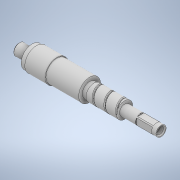
# Autodesk Inventor part: 75. Шестерня спидометра ведомая
Saved by Autodesk Inventor 2021 (Build 250183000, 183)
## iProperties
Created: 2021-03-27
Part Number: 75. Шестерня спидометра ведомая
Material: Типовые
Document SubType Name: Modeling
Designer: Данил
Density: 1 g/cm^3
Appearance: По умолчанию
Author: Данил
Autodesk Inventor part; units mm, degrees
ref_plane "YZ Plane" through (0, 0, 0) normal (1, 0, 0) x (0, 1, 0)
ref_plane "XZ Plane" through (0, 0, 0) normal (0, 1, 0) x (-1, 0, 0)
ref_plane "XY Plane" through (0, 0, 0) normal (0, 0, 1) x (1, 0, 0)
sketch "Эскиз1" plane through (0, 0, 0) normal (0, 0, 1) x (1, 0, 0)
  line L0 (-48.75, 0) -> (48.75, 0)
  line L1 (48.75, 0) -> (48.75, -3.5)
  line L2 (48.75, -3.5) -> (23.75, -3.5)
  line L3 (23.75, -3.5) -> (23.75, -5.5)
  line L4 (23.75, -5.5) -> (2.75, -5.5)
  line L5 (2.75, -5.5) -> (2.75, -5)
  line L6 (2.75, -5) -> (-0.25, -5)
  line L7 (-0.25, -5) -> (-0.25, -7.5)
  line L8 (-0.25, -7.5) -> (-22.75, -7.5)
  line L9 (-22.75, -7.5) -> (-22.75, -10.55)
  line L10 (-22.75, -10.55) -> (-36.75, -10.55)
  line L11 (-36.75, -10.55) -> (-36.75, -7.5)
  line L12 (-36.75, -7.5) -> (-39.75, -7.5)
  line L13 (-39.75, -7.5) -> (-39.75, -3.5)
  line L14 (-39.75, -3.5) -> (-41.25, -3.5)
  line L15 (-41.25, -3.5) -> (-41.25, -4)
  line L16 (-41.25, -4) -> (-48.25, -4)
  line L17 (-48.75, -3.5) -> (-48.75, 0)
  line L18 (-48.25, -4) -> (-48.75, -3.5)
  point P0 (0, 0)
  point P1 (0, 0)
  point P2 (-48.75, -4)
  dimension "d0" = 97.5
  dimension "d1" = 7
  dimension "d2" = 25
  dimension "d3" = 11
  dimension "d4" = 10
  dimension "d5" = 3
  dimension "d6" = 15
  dimension "d7" = 24
  dimension "d8" = 14
  dimension "d9" = 15
  dimension "d10" = 0.5
  dimension "d11" = 45
  dimension "d12" = 8
  dimension "d13" = 7
  dimension "d14" = 1.5
  dimension "d15" = 9
  dimension "d16" = 3
  dimension "d17" = 21.1
  constraints: 38 end point, 10 perpendicular, 6 vertical, 3 point on line, 2 coincident, 1 horizontal, 1 midpoint, 1 parallel
  measures "d0" distance of L0.start L0.end
  measures "d1" diameter of L2 L0
  measures "d2" horizontal distance of L0.end L2.end
  measures "d3" diameter of L4 L0
  measures "d4" diameter of L6 L0
  measures "d5" distance of L5.end L6.end
  measures "d6" diameter of L8 L0
  measures "d7" distance between parallel lines of L7 L3
  measures "d8" distance of L9.end L10.end
  measures "d9" diameter of L12 L0
  measures "d10" distance of L16.end point (-48.75, -4)
  measures "d11" angle of L16 L18
  measures "d12" diameter of L16 L0
  measures "d13" diameter of L14 L0
  measures "d14" distance of L13.end L14.end
  measures "d15" distance from line of L0.start L13
  measures "d16" distance of L11.end L12.end
  measures "d17" diameter of L10 L0
revolve "Вращение1" add sketch "Эскиз1" angle 360 about axis through (-48.75, 0, 0) along (1, 0, 0)
sketch "Эскиз2" plane through (0, 0, 0) normal (0, 0, 1) x (1, 0, 0)
  line L0 (48.75, 3.5) -> (23.75, 3.5) projected
  line L1 (48.75, 3.5) -> (48.75, -3.5) projected
  line L2 (48.75, 3.5) -> (45.85, 3.5)
  line L3 (45.65, 2.75) -> (34.85, 2.75)
  line L4 (34.75, 2.85) -> (34.75, 3.4)
  line L5 (45.75, 2.85) -> (45.75, 3.4)
  line L6 (34.65, 3.5) -> (23.75, 3.5)
  line L7 (23.75, 5.5) -> (23.75, -5.5) projected
  arc A0 (34.75, 3.4) -> (34.65, 3.5) centre (34.65, 3.4) ccw
  arc A1 (34.75, 2.85) -> (34.85, 2.75) centre (34.85, 2.85) ccw
  arc A2 (45.65, 2.75) -> (45.75, 2.85) centre (45.65, 2.85) ccw
  arc A3 (45.85, 3.5) -> (45.75, 3.4) centre (45.85, 3.4) ccw
  line L8 (23.75, 3.5) -> (48.75, 3.5)
  point P0 (0, 0)
  point P1 (45.75, 3.5)
  point P2 (45.75, 2.75)
  point P3 (34.75, 2.75)
  point P4 (34.75, 3.5)
  dimension "d19" = 3
  dimension "d20" = 14
  dimension "d21" = 0.75
  dimension "d22" = 0.1
  dimension "d23" = 0.1
  constraints: 12 end point, 10 point on line, 8 point on circle, 8 tangent, 4 centre point, 2 equal radius, 2 perpendicular, 1 collinear, 1 horizontal, 1 vertical
  measures "d19" distance of L0.start point (45.75, 3.5)
  measures "d20" distance from line of point (34.75, 2.75) L1
  measures "d21" distance of point (45.75, 2.75) point (45.75, 3.5)
  measures "d22" radius of A0
  measures "d23" radius of A2
extrude "Выдавливание1" cut sketch "Эскиз2" against normal through all both and the other way through all
mirror "Зеркальное отражение1" about plane through (0, 0, 0) normal (0, 1, 0) of "Выдавливание1"
pattern_circular "Круговой массив1" count 2 over 90 about axis through (36.25, 0, 0) along (-1, 0, 0) of "Выдавливание1"
mirror "Зеркальное отражение2" about plane through (0, 0, 0) normal (0, 0, 1) of "Круговой массив1"
ref_plane "РабПлоскость1" through (23.75, 0, 5.5) normal (0.2255336, -0.9742354, 0) x (0.9742354, 0.2255336, 0)
sketch "Эскиз3" plane through (23.75, 0, 5.5) normal (0.2255336, -0.9742354, 0) x (0.9742354, 0.2255336, 0)
  line L0 (-0.6243, 0) -> (-0.2121, -0.4121)
  line L1 (0.6243, 0) -> (0.2121, -0.4121)
  arc A0 (-0.2121, -0.4121) -> (0.2121, -0.4121) centre (0, -0.2) ccw
  line L2 (-0.6243, 0) -> (0.6243, 0)
  point P0 (-23.1381, -5.5)
  point P1 (0, 0)
  point P2 (0, -0.5)
  dimension "d37" = 90
  dimension "d38" = 0.5
  dimension "d39" = 0.5
  dimension "d40" = 0.3
  constraints: 6 end point, 3 point on circle, 2 tangent, 2 vertical alignment, 1 centre point, 1 horizontal alignment
  measures "d37" angle of L0 L1
  measures "d38" vertical distance of point (0, -0.5) L1.start
  measures "d39" vertical distance of point (0, -0.5) L0.start
  measures "d40" radius of A0
sketch3d "3D эскиз1"
  helix H0 starts at (3.75, 0, -5.5) axis through (3.75, 0, 0) along (1, 0, 0) pitch 8 turns 2.5 hand right
sweep "Сдвиг1" cut profiles "Эскиз3" path "3D эскиз1"
sketch "Эскиз4" plane through (48.75, 0, 0) normal (1, 0, 0) x (0, 0, -1)
  circle A0 centre (0, 0) radius 3.5 projected
  point P0 (0, 0)
hole "Отверстие1" at (48.75, 0, 0) direction (-1, 0, 0) diameter 4 depth 27 tip angle 120 counterbore diameter 5 counterbore depth 3
chamfer "Фаска1" distance 0.5 angle 60 1 edges at (48.75, 0, 2.5) measured on face at (48.75, 0, 3)
sketch "Эскиз5" plane through (0, 0, 0) normal (0, 0, 1) x (1, 0, 0)
  line L0 (-36.75, 10.55) -> (-36.75, -10.55) projected
  line L1 (-22.75, 10.55) -> (-22.75, -10.55) projected
  line L2 (-36.75, 10.55) -> (-22.75, 10.55)
  line L3 (-22.75, 10.55) -> (-22.75, 8)
  line L4 (-22.75, 8) -> (-36.75, 8)
  line L5 (-36.75, 8) -> (-36.75, 10.55)
  line L6 (-36.75, 0) -> (-22.75, 0)
  point P0 (0, 0)
  dimension "d53" = 16
  constraints: 10 end point, 2 midpoint, 2 parallel, 1 horizontal, 1 perpendicular, 1 point on line
  measures "d53" diameter of L4 L6
revolve "Вращение2" cut sketch "Эскиз5" angle 360 about axis through (-36.75, 0, 0) along (1, 0, 0) contours L2 L1 L4 L0
